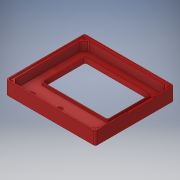
# Autodesk Inventor part: case front
Saved by Autodesk Inventor 2018 (Build 220112000, 112)
## iProperties
Created: 2017-11-13
Part Number: case front
Material: ABS-Kunststoff
Document SubType Name: Modeling
Designer: tillm
Density: 1.06 g/cm^3
Appearance: Rot
Author: tillm
Autodesk Inventor part; units mm, degrees
ref_plane "YZ Plane" through (0, 0, 0) normal (1, 0, 0) x (0, 1, 0)
ref_plane "XZ Plane" through (0, 0, 0) normal (0, 1, 0) x (-1, 0, 0)
ref_plane "XY Plane" through (0, 0, 0) normal (0, 0, 1) x (1, 0, 0)
sketch "Skizze1" plane through (0, 0, 0) normal (0, 0, 1) x (1, 0, 0)
  line L0 (-52.3, 47.7) -> (52.3, 47.7)
  line L1 (54.3, 45.7) -> (54.3, -45.7)
  line L2 (52.3, -47.7) -> (-52.3, -47.7)
  line L3 (-54.3, -45.7) -> (-54.3, 45.7)
  line L4 (-54.3, 47.7) -> (54.3, -47.7) construction
  line L5 (54.3, 47.7) -> (-54.3, -47.7) construction
  arc A0 (-52.3, 47.7) -> (-54.3, 45.7) centre (-52.3, 45.7) ccw
  arc A1 (54.3, 45.7) -> (52.3, 47.7) centre (52.3, 45.7) ccw
  arc A2 (-54.3, -45.7) -> (-52.3, -47.7) centre (-52.3, -45.7) ccw
  arc A3 (52.3, -47.7) -> (54.3, -45.7) centre (52.3, -45.7) ccw
  point P0 (0, 0)
  dimension "d0" = 108.6
  dimension "d1" = 95.4
  dimension "d2" = 2
  constraints: 12 end point, 8 point on circle, 8 point on line, 8 tangent, 4 centre point, 3 equal radius, 2 midpoint, 2 parallel, 1 horizontal, 1 perpendicular
  measures "d0" distance of L4.end L5.end
  measures "d1" distance of L5.start L4.end
  measures "d2" radius of A0
extrude "Extrusion1" add sketch "Skizze1" along normal blind 16
shell "Wandung1" thickness 3 removed faces 1 at (17.4333, -15.9, 16)
sketch "Skizze2" plane through (0, 0, 0) normal (0, 0, -1) x (-1, 0, 0)
  line L0 (39.4, 33.7) -> (-39.4, 33.7)
  line L1 (-39.4, 33.7) -> (-39.4, -18.1)
  line L2 (-39.4, -18.1) -> (39.4, -18.1)
  line L3 (39.4, -18.1) -> (39.4, 33.7)
  line L4 (-52.3, 47.7) -> (52.3, 47.7) projected
  line L5 (54.3, 45.7) -> (54.3, -45.7) projected
  circle A0 centre (36.3, -35.4) radius 4
  line L6 (3.45, -32.9) -> (3.45, -37.9) construction
  line L7 (0.45, -32.9) -> (0.45, -37.9)
  line L8 (6.45, -37.9) -> (6.45, -32.9)
  arc A1 (6.45, -32.9) -> (0.45, -32.9) centre (3.45, -32.9) ccw
  arc A2 (0.45, -37.9) -> (6.45, -37.9) centre (3.45, -37.9) ccw
  point P0 (0, 0)
  point P1 (3.45, -35.4)
  dimension "d6" = 14
  dimension "d7" = 14.9
  dimension "d8" = 78.8
  dimension "d9" = 51.8
  dimension "d10" = 8
  dimension "d11" = 18
  dimension "d12" = 17.3
  dimension "d13" = 6
  dimension "d14" = 0
  dimension "d15" = 5
  dimension "d16" = 29.85
  constraints: 16 end point, 4 point on circle, 4 tangent, 3 centre point, 3 parallel, 1 horizontal, 1 midpoint, 1 perpendicular, 1 vertical
  measures "d6" distance between parallel lines of L4 L0
  measures "d7" distance between parallel lines of L5 L3
  measures "d8" distance of L1.end L2.end
  measures "d9" distance between parallel lines of L0 L2
  measures "d10" diameter of A0
  measures "d11" distance from line of L5 A0.centre
  measures "d12" distance from line of A0.centre L2
  measures "d13" diameter of A2
  measures "d14" vertical distance of A0.centre point (3.45, -35.4)
  measures "d15" distance of L6.start L6.end
  measures "d16" distance from line of A0.centre L8
extrude "Extrusion2" cut sketch "Skizze2" against normal through all
sketch "Skizze3" plane through (-51.3, -44.7, 3) normal (0, 0, 1) x (1, 0, 0)
  line L0 (90.7, 26.6) -> (11.9, 26.6) projected
  line L1 (11.9, 26.6) -> (11.9, 78.4) projected
  line L2 (11.9, 78.4) -> (90.7, 78.4) projected
  line L3 (90.7, 78.4) -> (90.7, 26.6) projected
  line L4 (11.9, 78.4) -> (90.7, 26.6) construction
  line L5 (90.7, 78.4) -> (11.9, 26.6) construction
  line L6 (10.7, 79.6) -> (91.9, 79.6)
  line L7 (91.9, 79.6) -> (91.9, 25.4)
  line L8 (91.9, 25.4) -> (10.7, 25.4)
  line L9 (10.7, 25.4) -> (10.7, 79.6)
  line L10 (10.7, 79.6) -> (91.9, 25.4) construction
  line L11 (91.9, 79.6) -> (10.7, 25.4) construction
  point P0 (51.3, 44.7)
  point P1 (51.3, 52.5)
  dimension "d19" = 1.2
  dimension "d20" = 1.2
  constraints: 16 end point, 3 midpoint, 2 parallel, 1 horizontal, 1 perpendicular
  measures "d19" distance between parallel lines of L2 L6
  measures "d20" distance between parallel lines of L3 L7
extrude "Extrusion3" add sketch "Skizze3" along normal blind 3
sketch "Skizze4" plane through (54.3, -45.7, 0) normal (1, 0, 0) x (0, 0, -1)
  line L0 (-16, 90.4) -> (-16, 1) projected
  line L1 (-16, 37.5) -> (-14.5, 37.5)
  line L2 (-14.5, 37.5) -> (-14.5, 68.7)
  line L3 (-14.5, 68.7) -> (-16, 68.7)
  line L4 (-16, 68.7) -> (-16, 37.5)
  line L5 (0, -2) -> (-16, -2) projected
  point P0 (0, 45.7)
  dimension "d23" = 1.5
  dimension "d24" = 39.5
  dimension "d25" = 31.2
  constraints: 8 end point, 2 parallel, 1 horizontal, 1 perpendicular, 1 point on line
  measures "d23" distance of L3.end L2.end
  measures "d24" distance between parallel lines of L5 L1
  measures "d25" distance of L1.end L2.end
extrude "Extrusion4" cut sketch "Skizze4" against normal up to next
chamfer "Fase1" distance 5 angle 45 4 edges at (-51.3, 44.7, 9.5) (51.3, 44.7, 9.5) (51.3, -44.7, 9.5) (-51.3, -44.7, 9.5)
sketch "Skizze6" plane through (0, 0, 16) normal (0, 0, 1) x (1, 0, 0)
  circle A0 centre (-50.8, 44.2) radius 1.5
  line L0 (52.3, 47.7) -> (-52.3, 47.7) projected
  line L1 (-54.3, 45.7) -> (-54.3, -45.7) projected
  circle A1 centre (50.8, 44.2) radius 1.5
  circle A2 centre (-50.8, -44.2) radius 1.5
  line L2 (-52.3, -47.7) -> (52.3, -47.7) projected
  circle A3 centre (50.8, -44.2) radius 1.5
  line L3 (54.3, 23) -> (54.3, 45.7) projected
  line L4 (54.3, -45.7) -> (54.3, -8.2) projected
  point P0 (0, 0)
  dimension "d41" = 3
  dimension "d42" = 3.5
  dimension "d43" = 3.5
  dimension "d44" = 3
  dimension "d45" = 3
  dimension "d46" = 3.5
  dimension "d47" = 3
  dimension "d48" = 3.5
  dimension "d49" = 3.5
  dimension "d50" = 3.5
  dimension "d51" = 3.5
  dimension "d52" = 3.5
  constraints: 4 centre point
  measures "d41" diameter of A0
  measures "d42" distance from line of L0 A0.centre
  measures "d43" distance from line of L1 A0.centre
  measures "d44" diameter of A1
  measures "d45" diameter of A2
  measures "d46" distance from line of L2 A2.centre
  measures "d47" diameter of A3
  measures "d48" distance from line of L0 A1.centre
  measures "d49" distance from line of L3 A1.centre
  measures "d50" distance from line of L4 A3.centre
  measures "d51" distance from line of L2 A3.centre
  measures "d52" distance from line of L1 A2.centre
extrude "Extrusion6" cut sketch "Skizze6" against normal blind 10
sketch "Skizze7" plane through (0, 0, 16) normal (0, 0, 1) x (1, 0, 0)
  line L0 (-53.1, -46.5) -> (53.1, -46.5)
  line L1 (53.1, -46.5) -> (53.1, 46.5)
  line L2 (53.1, 46.5) -> (-53.1, 46.5)
  line L3 (-53.1, 46.5) -> (-53.1, -46.5)
  line L4 (-53.1, -46.5) -> (53.1, 46.5) construction
  line L5 (53.1, -46.5) -> (-53.1, 46.5) construction
  line L6 (52.3, 47.7) -> (-52.3, 47.7) projected
  line L7 (54.3, 23) -> (54.3, 45.7) projected
  point P0 (0, 0)
  dimension "d55" = 1.2
  dimension "d56" = 1.2
  constraints: 12 end point, 2 midpoint, 2 parallel, 1 horizontal, 1 perpendicular
  measures "d55" distance between parallel lines of L2 L6
  measures "d56" distance between parallel lines of L7 L1
extrude "Extrusion7" cut sketch "Skizze7" against normal blind 2
fillet "Rundung1" radius 2 20 edges at (-53.1, 46.5, 15) (53.1, 46.5, 15) (-53.1, -46.5, 15) (53.1, -46.5, 15) (46.3, 44.7, 8.5) (51.3, 39.7, 8.5) (51.3, -39.7, 8.5) (46.3, -44.7, 8.5) (-46.3, -44.7, 8.5) (-51.3, -39.7, 8.5) (-46.3, 44.7, 8.5) (-51.3, 39.7, 8.5) (-39.4, 33.7, 3) (39.4, 33.7, 3) (39.4, -18.1, 3) (-39.4, -18.1, 3) (-40.6, 34.9, 4.5) (40.6, 34.9, 4.5) (40.6, -19.3, 4.5) (-40.6, -19.3, 4.5)
fillet "Rundung1" radius 0.5 4 edges at (54.3, 23, 15.25) (53.1, 23, 15.25) (54.3, -8.2, 15.25) (53.1, -8.2, 15.25)
